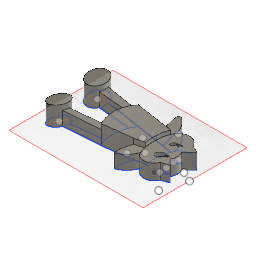
nekotaro (Autodesk Fusion 360 design; units mm, degrees)
Autodesk Fusion 360 part; units mm, degrees
sketch "スケッチ1" plane through (0, 0, 0) normal (0, 1, 0) x (1, 0, 0)
  line L0 (7, 1.5) -> (8, 1)
  line L1 (8, 1) -> (7, 0)
  line L2 (7, -1.5) -> (7.7098, -2.2098)
  line L3 (7.7098, -2.2098) -> (6.7394, -2.5434)
  arc A0 (7, -1.5) -> (7, 0) centre (5.7688, -0.75) ccw
  arc A1 (4.5, -3) -> (6.7394, -2.5434) centre (5.4755, -2.0646) ccw
  arc A2 (3.9615, -0.2975) -> (4.5, -3) centre (8.7627, -0.7458) ccw
  arc A3 (4.7214, 2.0292) -> (3.9615, -0.2975) centre (7.4426, -0.1469) ccw
  arc A4 (7, 1.5) -> (4.7214, 2.0292) centre (5.6579, 0.8916) ccw
  arc A5 (4.4351, 1.6124) -> (3, 4) centre (0.8237, 1.0669) ccw
  arc A6 (3, 4) -> (2.4696, 3.7328) centre (2.75, 3.8362) ccw
  arc A7 (2.4696, 3.7328) -> (3, 1.5) centre (21.0964, 6.9782) ccw
  line L4 (3, 1.5) -> (4.2766, 1.308)
  line L5 (3, 1.5) -> (-0.7213, 2.0596)
  arc A8 (2.7463, -2.0225) -> (2.4545, -4.257) centre (7.8275, -3.8223) ccw
  arc A9 (2.4545, -4.257) -> (4.1953, -2.2919) centre (1.5125, -1.6691) ccw
  line L6 (4.0336, -1.688) -> (2.7463, -2.0225)
  line L7 (2.7463, -2.0225) -> (-1, -2.5)
  arc A10 (-0.7213, 2.0596) -> (-1, -2.5) centre (2.6887, -0.4371) ccw
  ellipse E0 centre (-6.5, 2.5) end of major axis (-7.653, 2.1899) minor radius 1.5141
  line L8 (-5.347, 2.8101) -> (-7.653, 2.1899)
  line L9 (-6.8933, 3.9622) -> (-6.1067, 1.0378)
  ellipse E1 centre (-6.5, -2.5) end of major axis (-5.6937, -2.8339) minor radius 1.3081
  line L10 (-7.3063, -2.1661) -> (-5.6937, -2.8339)
  line L11 (-7.0005, -3.7085) -> (-5.9995, -1.2915)
  line L12 (-0.7213, 2.0596) -> (-5.347, 2.8101)
  line L13 (-5.4173, 1.6611) -> (-1.1794, 1.2659)
  line L14 (-1.3695, -1.6175) -> (-5.5524, -2.0809)
  line L15 (-5.6937, -2.8339) -> (-1, -2.5)
  ellipse E2 centre (5.5413, 0.3628) end of major axis (5.3748, 0.0685) minor radius 0.2124
  line L16 (5.7077, 0.657) -> (5.3748, 0.0685)
  line L17 (5.3564, 0.4673) -> (5.7261, 0.2582)
  ellipse E3 centre (5.8235, -1.688) end of major axis (5.4755, -2.0646) minor radius 0.4096
  line L18 (6.1714, -1.3114) -> (5.4755, -2.0646)
  line L19 (5.5226, -1.4101) -> (6.1243, -1.966)
  line L20 (5.7077, 0.657) -> (6.2756, 0.7903)
  line L21 (6.2756, 0.7903) -> (6.3934, 0.7237)
  line L22 (6.3934, 0.7237) -> (5.7733, 0.5781)
  line L23 (5.7893, 0.5044) -> (6.1, 0.5044)
  line L24 (6.1, 0.5044) -> (6.1874, 0.455)
  line L25 (6.1874, 0.455) -> (5.789, 0.455)
  line L26 (6.1714, -1.3114) -> (6.5, -1.2)
  line L27 (6.5, -1.2) -> (6.6475, -1.2557)
  line L28 (6.6475, -1.2557) -> (6.2367, -1.395)
  line L29 (6.2768, -1.5092) -> (6.5, -1.395)
  line L30 (6.5, -1.395) -> (6.6513, -1.4521)
  line L31 (6.6513, -1.4521) -> (6.2799, -1.6421)
  constraint perpendicular L1 L2
  constraint coincident A3 A5.start
  constraint coincident A3 L4.end
  constraint parallel L4 L5
  constraint coincident A2 A9.end
  constraint midpoint A2 L6.start
  constraint coincident E0 L8.start
  constraint coincident E0 L8.end
  constraint coincident E0 L9.start
  constraint coincident E0 L9.end
  constraint coincident E1 L10.start
  constraint coincident E1 L10.end
  constraint coincident E1 L11.start
  constraint coincident E1 L11.end
  constraint coincident E0 L13.start
  constraint coincident A10 L13.end
  constraint coincident A10 L14.start
  constraint coincident E1 L14.end
  constraint coincident E2 L16.start
  constraint coincident E2 L16.end
  constraint coincident E2 L17.start
  constraint coincident E2 L17.end
  constraint coincident E3 L18.start
  constraint coincident A1.centre E3
  constraint coincident E3 L19.start
  constraint coincident E3 L19.end
  constraint perpendicular L16 L21
  constraint coincident E2 L22.end
  constraint parallel L20 L22
  constraint coincident E2 L23.start
  constraint horizontal L23
  constraint parallel L17 L24
  constraint coincident E2 L25.end
  constraint parallel L23 L25
  constraint coincident E3 L28.end
  constraint parallel L26 L28
  constraint coincident E3 L29.start
  constraint parallel L27 L30
  constraint coincident E3 L31.end
  constraint parallel L29 L31
extrude "押し出し15" add sketch "スケッチ1" along normal blind 2 contours L0 L1 L2 L3 A0 A1 A2 A3 A4
extrude "押し出し16" add sketch "スケッチ1" along normal blind 2.5 contours A2 A3 L4 L5 L6 L7 A10
extrude "押し出し17" add sketch "スケッチ1" along normal blind 1.8 contours A3 A5 A6 A7 L4
extrude "押し出し18" add sketch "スケッチ1" along normal blind 1.8 contours A2 A8 A9 L6
extrude "押し出し19" add sketch "スケッチ1" along normal blind 1.8 contours A10 E0 L12 L13
extrude "押し出し20" add sketch "スケッチ1" along normal blind 1.8 contours A10 E1 L14 L15
extrude "押し出し21" add sketch "スケッチ1" along normal blind 2.5 contours E0 L8 L9 | E0 L8 L9 | E0 L8 L9 | E0 L8 L9
extrude "押し出し22" add sketch "スケッチ1" along normal blind 2.5 contours E1 L10 L11 | E1 L10 L11 | E1 L10 L11 | E1 L10 L11
extrude "押し出し23" add sketch "スケッチ1" along normal blind 1.5 contours E2 L16 L17 | E2 L16 L17 | E2 L16 L17 | E2 L16 L17 | E2 L20 L21 L22 | E3 L18 L19 | E3 L18 L19 | E3 L18 L19 | E3 L18 L19 | E3 L29 L30 L31 | E3 L26 L27 L28
